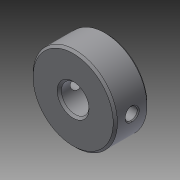
# Autodesk Inventor part: nylonClamp
Saved by Autodesk Inventor 2014 SP1 (Build 180222100, 222)
## iProperties
Created: 2014-11-10
Part Number: nylonClamp
Material: Generic
Document SubType Name: Modeling
Designer: rawrdong
Density: 1 g/cm^3
Appearance: Default
Author: rawrdong
Autodesk Inventor part; units mm, degrees
ref_plane "YZ Plane" through (0, 0, 0) normal (1, 0, 0) x (0, 1, 0)
ref_plane "XZ Plane" through (0, 0, 0) normal (0, 1, 0) x (-1, 0, 0)
ref_plane "XY Plane" through (0, 0, 0) normal (0, 0, 1) x (1, 0, 0)
sketch "Sketch1" plane through (0, 0, 0) normal (0, 1, 0) x (-1, 0, 0)
  circle A0 centre (0, 0) radius 3.275
  circle A1 centre (0, 0) radius 10
  dimension "d0" = 6.55
  dimension "d1" = 20
  constraints: 2 centre point, 2 coincident
  measures "d0" diameter of A0
  measures "d1" diameter of A1
extrude "Extrusion1" add sketch "Sketch1" along normal blind 8
chamfer "Chamfer1" distance 0.5 angle 45 4 edges at (10, 8, 0) (10, 0, 0) (3.275, 0, 0) (3.275, 8, 0)
sketch "Sketch2" plane through (0, 0, 0) normal (1, 0, 0) x (0, 1, 0)
  circle A0 centre (4, 0) radius 1.425
  line L0 (8, 3.275) -> (8, -3.275) projected
  line L1 (0, -3.275) -> (0, 3.275) projected
  line L2 (0, 0) -> (8, 0) construction
  dimension "d7" = 2.85
  constraints: 2 end point, 2 midpoint, 1 centre point, 1 horizontal alignment
  measures "d7" diameter of A0
extrude "Extrusion2" cut sketch "Sketch2" along normal through all both and the other way through all
chamfer "Chamfer2" distance 0.25 angle 45 3 edges at (-9.8979, 4.0001, 1.425) (-9.8979, 4, -1.425) (10, 2.5751, -0.0175)
body "Solid1"
